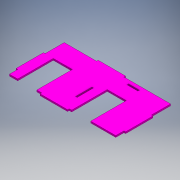
# Autodesk Inventor part: Celda celdas
Saved by Autodesk Inventor 2018 (Build 220112000, 112)
## iProperties
Created: 2020-03-11
Part Number: Celda celdas
Material: Madera (roble)
Document SubType Name: Modeling
Designer: joser
Density: 0.76 g/cm^3
Appearance: Magenta
Author: joser
Autodesk Inventor part; units mm, degrees
ref_plane "YZ Plane" through (0, 0, 0) normal (1, 0, 0) x (0, 1, 0)
ref_plane "XZ Plane" through (0, 0, 0) normal (0, 1, 0) x (-1, 0, 0)
ref_plane "XY Plane" through (0, 0, 0) normal (0, 0, 1) x (1, 0, 0)
sketch "Boceto1" plane through (0, 0, 0) normal (0, 0, 1) x (1, 0, 0)
  line L0 (0, 65) -> (-3, 65)
  line L1 (-3, 65) -> (-3, 15)
  line L2 (-3, 15) -> (0, 15)
  line L3 (0, 0) -> (0, 15)
  line L4 (0, 65) -> (0, 100)
  line L5 (194, 65) -> (197, 65)
  line L6 (197, 65) -> (197, 15)
  line L7 (197, 15) -> (194, 15)
  line L8 (194, 100) -> (194, 65)
  line L9 (194, 15) -> (194, 0)
  line L10 (15, 0) -> (15, 65)
  line L11 (15, 65) -> (50, 65)
  line L12 (50, 65) -> (50, 0)
  line L13 (15, 0) -> (0, 0)
  line L14 (113.5, 0) -> (113.5, 65)
  line L15 (113.5, 65) -> (148.5, 65)
  line L16 (148.5, 65) -> (148.5, 0)
  line L17 (194, 0) -> (148.5, 0)
  line L18 (95.5, 55) -> (98.5, 55)
  line L19 (98.5, 55) -> (98.5, 25)
  line L20 (98.5, 25) -> (95.5, 25)
  line L21 (95.5, 25) -> (95.5, 55)
  line L22 (59, 100) -> (59, 103)
  line L23 (59, 103) -> (109, 103)
  line L24 (109, 103) -> (109, 100)
  line L25 (0, 100) -> (59, 100)
  line L26 (109, 100) -> (194, 100)
  line L27 (109, 100) -> (209, 100) construction
  line L28 (59, 0) -> (59, -3)
  line L29 (59, -3) -> (109, -3)
  line L30 (109, -3) -> (109, 0)
  line L31 (113.5, 0) -> (109, 0)
  line L32 (59, 0) -> (50, 0)
  dimension "d0" = 194
  dimension "d1" = 100
  dimension "d3" = 50
  dimension "d8" = 3
  dimension "d13" = 35
  dimension "d14" = 65
  dimension "d15" = 15
  dimension "d16" = 3
  dimension "d17" = 30
  dimension "d19" = 95.5
  dimension "d20" = 15
  dimension "d23" = 15
  dimension "d24" = 3
  dimension "d25" = 50
  dimension "d26" = 88
  dimension "d28" = 3
  dimension "d29" = 25
  constraints: 66 end point, 22 perpendicular, 18 parallel, 8 collinear, 6 horizontal, 5 equal length, 4 vertical, 1 coincident
  measures "d0" distance of L9.end L3.start
  measures "d1" distance of L8.start L9.end
  measures "d3" distance of L0.end L1.end
  measures "d8" distance between parallel lines of L4 L1
  measures "d13" distance between parallel lines of L12 L10
  measures "d14" distance between parallel lines of L13 L11
  measures "d15" distance between parallel lines of L3 L10
  measures "d16" distance of L19.end L20.end
  measures "d17" distance of L18.end L19.end
  measures "d19" distance between parallel lines of L21 L3
  measures "d20" distance between parallel lines of L14 L19
  measures "d23" distance between parallel lines of L13 L2
  measures "d24" distance of L22.start L22.end
  measures "d25" distance of L22.end L23.end
  measures "d26" distance between parallel lines of L6 L24
  measures "d28" distance of L28.start L28.end
  measures "d29" distance between parallel lines of L31 L20
extrude "Extrusión1" add sketch "Boceto1" along normal blind 3
sketch "Boceto3" plane through (0, 0, 3) normal (0, 0, 1) x (1, 0, 0)
  line L0 (124, 93.5) -> (144, 93.5)
  line L1 (144, 93.5) -> (144, 90.5)
  line L2 (144, 90.5) -> (124, 90.5)
  line L3 (124, 90.5) -> (124, 93.5)
  line L4 (148.5, 0) -> (194, 0) projected
  line L5 (194, 65) -> (194, 100) projected
  point P0 (0, 0)
  dimension "d44" = 20
  dimension "d45" = 3
  dimension "d46" = 90.5
  dimension "d47" = 50
  constraints: 8 end point, 2 parallel, 1 horizontal, 1 perpendicular
  measures "d44" distance of L1.end L2.end
  measures "d45" distance of L0.end L1.end
  measures "d46" distance between parallel lines of L4 L2
  measures "d47" distance between parallel lines of L5 L1
extrude "Extrusión4" cut sketch "Boceto3" against normal blind 3
